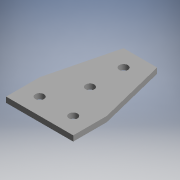
# Autodesk Inventor part: 25-4141
Saved by Autodesk Inventor 2017.3 (Build 213256000, 256)
## iProperties
Part Number: 25-4141
Material: Generic
Catalog Web Link: www.cadenas.de
Description: 25-4141, 25-4141-Black, 40-4341, 40-4341-Black-4 Hole Tee Joining Plate
Vendor: 8020
Document SubType Name: Modeling
Designer: partserver
Manufacturer: 8020
Mass: 11.9933 g
Surface Area: 72.2814 cm^2
Volume: 11.9933 cm^3
Density: 1 g/cm^3
Appearance: PSOLRGB-191-191-191
Category: PARTsolutions
Company: 8020
Title: 25-4141
Author: Cadenas PARTsolutions
Comments: 4 Hole Tee Joining Plate
PSOL_IDENT_0: {$CADENAS_DATA\23d-libs\8020\metric\joining_plates\25_4141.prj},194 {VTYP=3D},{NB=25-4141},{LINA=25-
PSOL_IDENT_1: 4141},{NN=25-4141, 25-4141-Black, 40-4341, 40-4341-Black},{DATE=31.07.2020 09:21:28},{GEOMDATE=16.01
PSOL_IDENT_2: .2019 16:00:00},{VERSION=},{LINEID=10},{WBVAR=},{WBNUMERIC=}  {NB=25-4141},{LINA=25-4141},{KT=DUMMY}
PSOL_IDENT_3: ,{PN=25-4141},{A=50.00},{B=75.00},{C=25.00},{D=25.00},{E=12.50},{F=6.35},{T=4.00},{W=.038},{A1=12.50
PSOL_IDENT_4: 00},{C1=37.500},{C2=12.500},{C3=62.500},{D1=4.000},{COLOR=.75,.75,.75}
NB: 25-4141
NN: 25-4141, 25-4141-Black, 40-4341, 40-4341-Black
NT: 4 Hole Tee Joining Plate
NBSYN: $PN.
LINA: 25-4141
CATALOG: 80/20
PN: 25-4141
A: 50
B: 75
C: 25
D: 25
E: 12.5
F: 6.35
T: 4
W: .038
SUPPLIER: 8020
ARTICLENO: 25-4141
BOMINFO: 25-4141
CREATOR: CADENAS GmbH
Autodesk Inventor part; units mm, degrees
ref_plane "YZ Plane" through (0, 0, 0) normal (1, 0, 0) x (0, 1, 0)
ref_plane "XZ Plane" through (0, 0, 0) normal (0, 1, 0) x (-1, 0, 0)
ref_plane "XY Plane" through (0, 0, 0) normal (0, 0, 1) x (1, 0, 0)
sketch "Sketch_1" plane through (0, 0, 0) normal (0, 0, 1) x (1, 0, 0)
  line L0 (-25, 25) -> (-25, 0)
  line L1 (-25, 0) -> (25, 0)
  line L2 (25, 0) -> (25, 25)
  line L3 (25, 25) -> (12.5, 75)
  line L4 (12.5, 75) -> (-12.5, 75)
  line L5 (-12.5, 75) -> (-25, 25)
  circle A0 centre (12.5, 12.5) radius 3.175
  circle A1 centre (0, 37.5) radius 3.175
  circle A2 centre (0, 62.5) radius 3.175
  circle A3 centre (-12.5, 12.5) radius 3.175
  constraints: 12 end point, 4 centre point
extrude "Extrusion1" add sketch "Sketch_1" along normal blind 4
body "Solid1"
